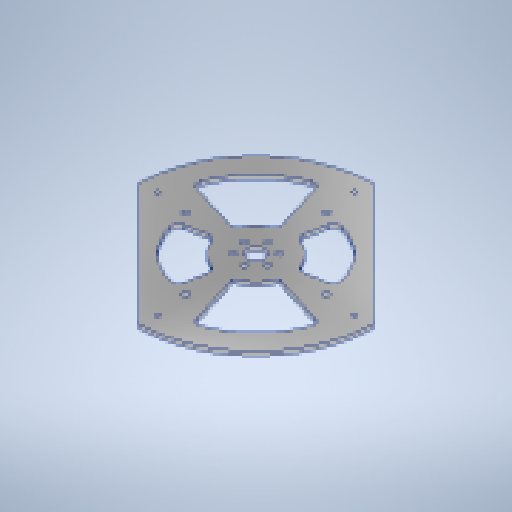
# Autodesk Inventor part: baseplate_R2toR3
Saved by Autodesk Inventor 2024.3 (Build 283343010, 343A)
## iProperties
Created: 2025-05-25
Part Number: baseplate_R2toR3
Material: アルミニウム 6061
Document SubType Name: Modeling
Designer: kshau
Density: 2.7 g/cm^3
Appearance: アルミニウム - フラット
Mass: 150.999 g
Surface Area: 394.685 cm^2
Volume: 55.9256 cm^3
Author: kshau
Autodesk Inventor part; units mm, degrees
ref_plane "YZ Plane" through (0, 0, 0) normal (1, 0, 0) x (0, 1, 0)
ref_plane "XZ Plane" through (0, 0, 0) normal (0, 1, 0) x (-1, 0, 0)
ref_plane "XY Plane" through (0, 0, 0) normal (0, 0, 1) x (1, 0, 0)
sketch "スケッチ1" plane through (0, 0, 0) normal (0, 1, 0) x (-1, 0, 0)
  circle A0 centre (0, 0) radius 86.2565
  circle A1 centre (0, 0) radius 6.25
  dimension "d0" = 172.513
  dimension "d1" = 12.5
  constraints: 2 centre point, 2 coincident
  measures "d0" diameter of A0
  measures "d1" diameter of A1
extrude "押し出し1" add sketch "スケッチ1" along normal blind 3
sketch "スケッチ2" plane through (0, 3, 0) normal (0, 1, 0) x (1, 0, 0)
  circle A0 centre (0, 0) radius 50.75
  point P0 (0, 50.75)
  point P1 (-50.75, 0)
  point P2 (0, -50.75)
  point P3 (50.75, 0)
  dimension "d4" = 101.5
  dimension "d7" = 360
  constraints: 1 coincident, 1 vertical alignment, 7 other
hole "穴1" at (0, 3, -50.75) at (-50.75, 3, 0) at (0, 3, 50.75) at (50.75, 3, 0) direction (0, -1, 0) diameter 4.3 end through all
sketch "スケッチ3" plane through (0, 3, 0) normal (0, 1, 0) x (1, 0, 0)
  line L0 (0, 0) -> (86.2565, 0)
  circle A0 centre (0, 0) radius 86.2565 projected
  circle A1 centre (0, 0) radius 6.25 projected
  line L1 (0, 0) -> (60.9926, -60.9926)
  line L2 (1.0606, -86.25) -> (-86.25, 1.0606)
  line L3 (86.25, -1.0606) -> (-1.0606, 86.25)
  point P0 (-1.0606, 86.25)
  point P1 (85.1894, 0)
  point P2 (86.25, -1.0606)
  dimension "d16" = 45
  dimension "d17" = 60.238
  constraints: 8 end point, 4 point on circle, 2 symmetric about line, 1 horizontal, 1 parallel
  measures "d16" angle of L0 L1
  measures "d17" distance between parallel lines of L1 L2
extrude "押し出し2" cut sketch "スケッチ3" against normal blind 3 contours L3 A0 L0 | L0 A0 L3 | A0 L2
sketch "スケッチ4" plane through (0, 3, 0) normal (0, 1, 0) x (1, 0, 0)
  circle A0 centre (0, 0) radius 6.25 projected
  circle A1 centre (0, 0) radius 12
  line L0 (0, 0) -> (-8.4853, -8.4853)
  line L1 (0, 0) -> (-12, 0)
  point P0 (3.1058, -11.5911)
  point P1 (11.5911, -3.1058)
  point P2 (8.4853, 8.4853)
  point P3 (-3.1058, 11.5911)
  point P4 (-11.5911, 3.1058)
  dimension "d20" = 24
  dimension "d21" = 45
  dimension "d24" = 360
  constraints: 4 end point, 2 coincident, 2 point on circle, 1 centre point, 1 horizontal, 7 other
  measures "d20" diameter of A1
  measures "d21" angle of L1 L0
hole "穴2" at (-8.4853, 3, 8.4853) at (3.1058, 3, 11.5911) at (11.5911, 3, 3.1058) at (8.4853, 3, -8.4853) at (-3.1058, 3, -11.5911) at (-11.5911, 3, -3.1058) direction (0, -1, 0) diameter 4.3 end through all
sketch "スケッチ5" plane through (0, 3, 0) normal (0, 1, 0) x (1, 0, 0)
  arc A0 (1.0606, -86.25) -> (86.25, -1.0606) centre (0, 0) ccw projected
  line L0 (14.0562, -85.1035) -> (-85.1035, 14.0562)
  arc A1 (-1.0606, 86.25) -> (-86.25, 1.0606) centre (0, 0) ccw projected
  line L1 (-86.25, 1.0606) -> (1.0606, -86.25) projected
  line L2 (-14.0562, 85.1035) -> (85.1035, -14.0562)
  line L3 (86.25, -1.0606) -> (-1.0606, 86.25) projected
  line L4 (-86.25, 1.0606) -> (-1.0606, 86.25)
  line L5 (1.0606, -86.25) -> (86.25, -1.0606)
  line L6 (-73.8926, 2.8453) -> (-2.8453, 73.8926)
  line L7 (80.9636, 4.2257) -> (2.8453, -73.8926)
  point P0 (73.8926, -2.8453)
  dimension "d33" = 10
  dimension "d34" = 10
  dimension "d35" = 7.476
  dimension "d36" = 7.476
  constraints: 12 end point, 6 point on line, 4 perpendicular, 4 point on circle, 3 coincident, 2 parallel
  measures "d33" distance between parallel lines of L1 L0
  measures "d34" distance between parallel lines of L3 L2
  measures "d35" distance between parallel lines of L4 L6
  measures "d36" distance between parallel lines of L5 L7
hole "穴3" at (-73.8926, 3, -2.8453) at (-2.8453, 3, -73.8926) at (73.8926, 3, 2.8453) at (2.8453, 3, 73.8926) direction (0, -1, 0) diameter 3.2 end through all
sketch "スケッチ6" plane through (0, 3, 0) normal (0, 1, 0) x (1, 0, 0)
  circle A0 centre (0, 0) radius 6.25 projected
  circle A1 centre (0, 0) radius 70
  circle A2 centre (0, 0) radius 50
  circle A3 centre (-2.8453, 73.8926) radius 1.6 projected
  line L0 (0, 0) -> (-2.8453, 73.8926)
  circle A4 centre (-73.8926, 2.8453) radius 1.6 projected
  line L1 (0, 0) -> (-73.8926, 2.8453)
  line L2 (0, 0) -> (-20.7056, 66.8676)
  line L3 (0, 0) -> (-66.8676, 20.7056)
  circle A5 centre (0, 0) radius 25
  circle A6 centre (0, 50.75) radius 2.15 projected
  line L4 (0, 0) -> (0, 50.75)
  line L5 (0, 0) -> (8.6824, 49.2404)
  line L6 (0, 0) -> (49.2404, 8.6824)
  circle A7 centre (50.75, 0) radius 2.15 projected
  line L7 (0, 0) -> (50.75, 0)
  line L8 (0, 0) -> (-49.2404, -8.6824)
  line L9 (0, 0) -> (-8.6824, -49.2404)
  line L10 (0, 0) -> (20.7056, -66.8676)
  line L11 (0, 0) -> (66.8676, -20.7056)
  circle A8 centre (0, 0) radius 40
  point P0 (-4.3412, -24.6202)
  point P1 (-24.6202, -4.3412)
  point P2 (47.7626, -14.7897)
  point P3 (23.8813, -7.3948)
  point P4 (7.3948, -23.8813)
  point P5 (14.7897, -47.7626)
  point P6 (24.6202, 4.3412)
  point P7 (4.3412, 24.6202)
  point P8 (-23.8813, 7.3948)
  point P9 (-7.3948, 23.8813)
  point P10 (-14.7897, 47.7626)
  point P11 (-47.7626, 14.7897)
  point P12 (66.8676, -20.7056)
  point P13 (20.7056, -66.8676)
  point P14 (38.2101, -11.8318)
  point P15 (11.8318, -38.2101)
  point P16 (-38.2101, 11.8318)
  point P17 (-11.8318, 38.2101)
  dimension "d44" = 140
  dimension "d45" = 100
  dimension "d46" = 15
  dimension "d47" = 15
  dimension "d48" = 50
  dimension "d49" = 10
  dimension "d50" = 10
  dimension "d53" = 360
  dimension "d57" = 80
  constraints: 24 end point, 5 coincident, 4 centre point, 4 point on circle, 1 horizontal, 1 vertical, 21 other
  measures "d44" diameter of A1
  measures "d45" diameter of A2
  measures "d46" angle of L0 L2
  measures "d47" angle of L1 L3
  measures "d48" diameter of A5
  measures "d49" angle of L4 L5
  measures "d50" angle of L7 L6
  measures "d57" diameter of A8
extrude "押し出し3" cut sketch "スケッチ6" against normal blind 10 contours A5 L5 A8 L6 | L11 A8 L10 A5 | A8 L5 A2 L6 | L11 A2 L10 A8 | A5 L3 A8 L2 | A5 L9 A8 L8 | L11 A1 L10 A2 | A8 L3 A2 L2 | A8 L9 A2 L8 | A2 L3 A1 L2
fillet "フィレット1" radius 5 14 edges at (-20.7056, 1.5, -66.8676) (-66.8676, 1.5, -20.7056) (-49.2404, 1.5, 8.6824) (-24.6202, 1.5, 4.3412) (-8.6824, 1.5, 49.2404) (-4.3412, 1.5, 24.6202) (20.7056, 1.5, 66.8676) (66.8676, 1.5, 20.7056) (24.6202, 1.5, -4.3412) (49.2404, 1.5, -8.6824) (8.6824, 1.5, -49.2404) (4.3412, 1.5, -24.6202) (-7.3948, 1.5, -23.8813) (-23.8813, 1.5, -7.3948)
